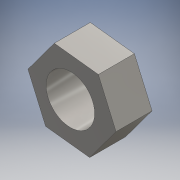
# Autodesk Inventor part: nut_5_mm
Saved by Autodesk Inventor 2016 (Build 200138000, 138)
## iProperties
Created: 2017-01-05
Part Number: nut_5_mm
Material: Generic
Document SubType Name: Modeling
Designer: hesaon
Density: 1 g/cm^3
Appearance: Default
Author: hesaon
Autodesk Inventor part; units mm, degrees
ref_plane "YZ Plane" through (0, 0, 0) normal (1, 0, 0) x (0, 1, 0)
ref_plane "XZ Plane" through (0, 0, 0) normal (0, 1, 0) x (-1, 0, 0)
ref_plane "XY Plane" through (0, 0, 0) normal (0, 0, 1) x (1, 0, 0)
sketch "Sketch1" plane through (0, 0, 0) normal (0, 1, 0) x (-1, 0, 0)
  circle A0 centre (0.1666, 0) radius 2.5
  line L0 (2.7166, -3.671) -> (-1.8209, -4.1881)
  line L1 (-1.8209, -4.1881) -> (-4.5375, -0.5171)
  line L2 (-4.5375, -0.5171) -> (-2.7166, 3.671)
  line L3 (-2.7166, 3.671) -> (1.8209, 4.1881)
  line L4 (1.8209, 4.1881) -> (4.5375, 0.5171)
  line L5 (4.5375, 0.5171) -> (2.7166, -3.671)
  point P0 (0, 0)
  point P1 (0, 0)
  dimension "d0" = 5
  dimension "d1" = 7.91
  constraints: 12 end point, 1 centre point, 1 coincident, 13 other
  measures "d0" diameter of A0
  measures "d1" distance between parallel lines of L2 L5
extrude "Extrusion1" add sketch "Sketch1" along normal blind 3.71
body "Solid1"
